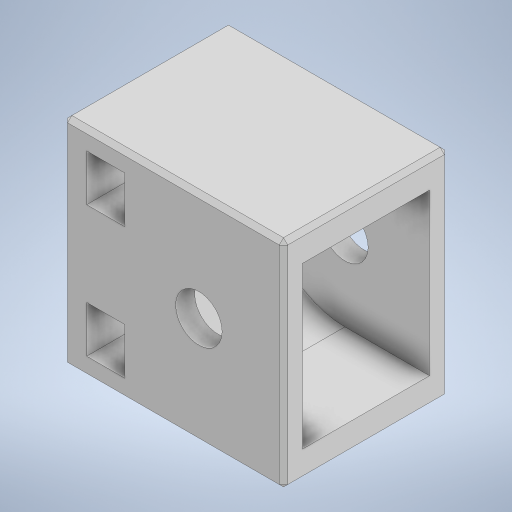
# Autodesk Inventor part: X-End-Floating-Idler v0.1
Saved by Autodesk Inventor 2023 (Build 270158000, 158)
## iProperties
Created: 2023-07-26
Part Number: X-End-Floating-Idler v0.1
Material: Generic
Document SubType Name: Modeling
Designer: Parker
Density: 1 g/cm^3
Appearance: Default
Author: Parker
Autodesk Inventor part; units mm, degrees
ref_plane "YZ Plane" through (0, 0, 0) normal (1, 0, 0) x (0, 1, 0)
ref_plane "XZ Plane" through (0, 0, 0) normal (0, 1, 0) x (-1, 0, 0)
ref_plane "XY Plane" through (0, 0, 0) normal (0, 0, 1) x (1, 0, 0)
sketch "Sketch1" plane through (0, 0, 0) normal (0, 0, 1) x (1, 0, 0)
  circle A0 centre (0, 0) radius 6
  line L0 (-10, -12.75) -> (10, -12.75)
  line L1 (10, -12.75) -> (10, 12.75)
  line L2 (10, 12.75) -> (-10, 12.75)
  line L3 (-10, 12.75) -> (-10, -12.75)
  line L4 (-10, -12.75) -> (10, 12.75) construction
  line L5 (10, -12.75) -> (-10, 12.75) construction
  line L6 (-10, -12.75) -> (-16, -12.75)
  line L7 (-16, -12.75) -> (-16, 12.75)
  line L8 (-16, 12.75) -> (-10, 12.75)
  line L9 (-10, 12.75) -> (-10, -12.75)
  dimension "d0" = 12
  dimension "d1" = 25.5
  dimension "d2" = 20
  dimension "d20" = 6
  constraints: 20 end point, 4 parallel, 2 horizontal, 2 midpoint, 2 perpendicular, 1 centre point, 1 coincident, 1 point on line
  measures "d0" diameter of A0
  measures "d1" distance of L1.end L0.end
  measures "d2" distance of L1.end L2.end
  measures "d20" distance between parallel lines of L3 L7
extrude "Extrusion1" add sketch "Sketch1" along normal blind 19.5 contours A0 | L3 L2 L1 L0 | L6 L7 L8 L3
ref_plane "Work Plane1" through (0, 0, 9.75) normal (0, 0, 1) x (1, 0, 0)
sketch "Sketch2" plane through (0, 0, 9.75) normal (0, 0, 1) x (1, 0, 0)
  circle A0 centre (0, 0) radius 9.5
  line L0 (-10, -9.5) -> (10, -9.5)
  line L1 (10, -9.5) -> (10, 9.5)
  line L2 (10, 9.5) -> (-10, 9.5)
  line L3 (-10, 9.5) -> (-10, -9.5)
  line L4 (-10, -9.5) -> (10, 9.5) construction
  line L5 (10, -9.5) -> (-10, 9.5) construction
  point P0 (0, 9.5)
  point P1 (0, -9.5)
  dimension "d5" = 19
  dimension "d6" = 20
  dimension "d7" = 19
  constraints: 12 end point, 2 midpoint, 2 parallel, 1 centre point, 1 coincident, 1 horizontal, 1 perpendicular
  measures "d5" diameter of A0
  measures "d6" distance of L2.end L1.end
  measures "d7" distance of L1.end L0.end
extrude "Extrusion2" cut sketch "Sketch2" along normal mid plane 15 contours A0 | A0 L2 L1 L0
sketch "Sketch3" plane through (0, 0, 19.5) normal (0, 0, 1) x (1, 0, 0)
  point P0 (0, 0)
  point P1 (0, 0)
  constraints: 1 coincident
hole "Hole1" at (0, 0, 19.5) direction (0, 0, -1) diameter 5.5 end through all clearance for "Socket Head Cap Screw" size "M5" standard "Ansi Metric M Profile"
sketch "Sketch4" plane through (-16, -12.75, 0) normal (-1, 0, 0) x (0, 0, 1)
  line L0 (0, 25.5) -> (19.5, 25.5) projected
  line L1 (9.75, 25.5) -> (9.75, 0)
  line L2 (0, 0) -> (19.5, 0) projected
  point P0 (9.75, 20.5)
  point P1 (9.75, 5)
  dimension "d21" = 5
  dimension "d22" = 5
  constraints: 2 end point, 2 midpoint, 2 point on line
  measures "d21" distance from line of L0 point (9.75, 20.5)
  measures "d22" distance from line of L2 point (9.75, 5)
hole "Hole2" at (-16, 7.75, 9.75) at (-16, -7.75, 9.75) direction (1, 0, 0) diameter 3.4 depth 8 clearance for "Hex Head Machine Screw" size "M3" standard "Ansi Metric M Profile"
sketch "Sketch5" plane through (0, 0, 19.5) normal (0, 0, 1) x (1, 0, 0)
  line L0 (-16, 6.05) -> (-16, 9.45) projected
  line L1 (-8, 9.45) -> (-8, 6.05) projected
  line L2 (-16, -9.45) -> (-16, -6.05) projected
  line L3 (-8, -6.05) -> (-8, -9.45) projected
  line L4 (-16, 7.75) -> (-8, 7.75)
  line L5 (-16, -7.75) -> (-8, -7.75)
  line L6 (-13.25, 10.5) -> (-10.75, 10.5)
  line L7 (-10.75, 10.5) -> (-10.75, 5)
  line L8 (-10.75, 5) -> (-13.25, 5)
  line L9 (-13.25, 5) -> (-13.25, 10.5)
  line L10 (-13.25, 10.5) -> (-10.75, 5) construction
  line L11 (-10.75, 10.5) -> (-13.25, 5) construction
  line L12 (-13.25, -5) -> (-10.75, -5)
  line L13 (-10.75, -5) -> (-10.75, -10.5)
  line L14 (-10.75, -10.5) -> (-13.25, -10.5)
  line L15 (-13.25, -10.5) -> (-13.25, -5)
  line L16 (-13.25, -5) -> (-10.75, -10.5) construction
  line L17 (-10.75, -5) -> (-13.25, -10.5) construction
  point P0 (0, 0)
  point P1 (-12, 7.75)
  point P2 (-12, -7.75)
  dimension "d30" = 2.5
  dimension "d31" = 5.5
  dimension "d32" = 2.5
  dimension "d33" = 5.5
  constraints: 28 end point, 10 midpoint, 4 parallel, 2 horizontal, 2 perpendicular
  measures "d30" distance of L7.end L8.end
  measures "d31" distance of L6.end L7.end
  measures "d32" distance of L13.end L14.end
  measures "d33" distance of L12.end L13.end
extrude "Extrusion3" cut sketch "Sketch5" against normal blind 13
chamfer "Chamfer1" distance 2 angle 45 2 edges at (-10.75, 7.75, 19.5) (-10.75, -7.75, 19.5)
chamfer "Chamfer2" distance 0.5 angle 45 12 edges at (-16, 12.75, 9.75) (-16, 0, 0) (-16, -12.75, 9.75) (-16, 0, 19.5) (-3, 12.75, 19.5) (-3, 12.75, 0) (-3, -12.75, 0) (-3, -12.75, 19.5) (10, 0, 19.5) (10, 12.75, 9.75) (10, 0, 0) (10, -12.75, 9.75)
body "Solid1"
